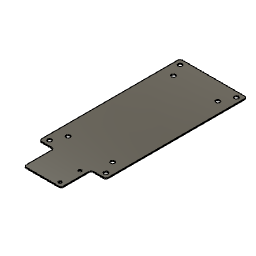
GAD Mount Plane v1 (Autodesk Fusion 360 design; units mm, degrees)
Autodesk Fusion 360 part; units mm, degrees
sketch "Sketch1" plane through (0, 0, 0) normal (0, 0, 1) x (1, 0, 0)
  line L0 (45, 95) -> (-45, 95)
  line L1 (-45, 95) -> (-45, -95)
  line L2 (-45, -95) -> (45, -95)
  line L3 (45, -95) -> (45, 95)
  line L4 (45, 95) -> (-45, -95) construction
  line L5 (-45, 95) -> (45, -95) construction
  line L6 (30, 71) -> (-30, 71) construction
  line L7 (-30, 71) -> (-30, -71) construction
  line L8 (-30, -71) -> (30, -71) construction
  line L9 (30, -71) -> (30, 71) construction
  line L10 (30, 71) -> (-30, -71) construction
  line L11 (-30, 71) -> (30, -71) construction
  circle A0 centre (-30, 71) radius 2.75
  circle A1 centre (30, 71) radius 2.75
  circle A2 centre (-30, -71) radius 2.75
  circle A3 centre (30, -71) radius 2.75
  line L12 (38, 88) -> (-38, 88) construction
  line L13 (-38, 88) -> (-38, -88) construction
  line L14 (-38, -88) -> (38, -88) construction
  line L15 (38, -88) -> (38, 88) construction
  line L16 (38, 88) -> (-38, -88) construction
  line L17 (-38, 88) -> (38, -88) construction
  circle A4 centre (38, 88) radius 2.75
  circle A5 centre (-38, 88) radius 2.75
  circle A6 centre (-38, -88) radius 2.75
  circle A7 centre (38, -88) radius 2.75
  line L18 (-25, -95) -> (25, -95)
  line L19 (25, -95) -> (25, -135.5)
  line L20 (25, -135.5) -> (-25, -135.5)
  line L21 (-25, -135.5) -> (-25, -95)
  line L22 (18, -130) -> (18, -103) construction
  circle A8 centre (18, -130) radius 2
  circle A9 centre (18, -103) radius 2
  line L23 (18, -116.5) -> (2.6311, -116.5) construction
  point P0 (0, -95)
  dimension "d1" = 76
  dimension "d2" = 176
  dimension "d3" = 190
  dimension "d4" = 90
  dimension "d5" = 142
  dimension "d6" = 60
  dimension "d7" = 27
  dimension "d8" = 15
  dimension "d9" = 50
  dimension "d12" = 12
  dimension "d13" = 19
  dimension "d14" = 4
  dimension "d15" = 5.5
  constraint horizontal L0
  constraint perpendicular L0 L1
  constraint parallel L0 L2
  constraint parallel L1 L3
  constraint coincident L4 origin
  constraint coincident L5 origin
  constraint horizontal L6
  constraint perpendicular L6 L7
  constraint parallel L6 L8
  constraint parallel L7 L9
  constraint coincident L10 origin
  constraint coincident L11 origin
  constraint coincident L6.end L7.start
  constraint coincident L6.start L9.end
  constraint coincident L7.end L8.start
  constraint coincident L8.end L9.start
  constraint horizontal L12
  constraint perpendicular L12 L13
  constraint parallel L12 L14
  constraint parallel L13 L15
  constraint coincident L16 origin
  constraint coincident L17 origin
  constraint coincident L12.start L15.end
  constraint coincident L12.end L13.start
  constraint coincident L13.end L14.start
  constraint coincident L14.end L15.start
  constraint horizontal L18
  constraint vertical L19
  constraint horizontal L20
  constraint vertical L21
  constraint coincident L2 L18.start
  constraint perpendicular L18 L22
  constraint coincident L22.start A8.centre
  constraint coincident L22.end A9.centre
  constraint equal A8 A9
  constraint equal A3 A7
  constraint equal A2 A3
  constraint equal A2 A6
  constraint equal A1 A3
  constraint equal A0 A1
  constraint equal A0 A5
  constraint equal A1 A4
  constraint midpoint L18 P0
  constraint midpoint L2 P0
  constraint midpoint L22 L23.start
  constraint perpendicular L22 L23
  measures "d1" distance of L12.start L12.end
  measures "d2" distance of L12.start L14.end
  measures "d3" distance of L0.start L2.end
  measures "d4" distance of L0.start L0.end
  measures "d5" distance of L6.start L8.end
  measures "d6" distance of L6.start L6.end
  measures "d7" distance of L22.start L22.end
  measures "d8" distance of L14 L22.end
  measures "d9" distance of L19.end L20.end
  measures "d12" distance of L9 L22
  measures "d13" distance of L20 L23
  measures "d14" diameter of A8
  measures "d15" diameter of A7
extrude "Extrude1" add sketch "Sketch1" along normal blind 1.27
fillet "Fillet1" radius 3 8 edges at (-25, -135.5, 0.635) (-25, -95, 0.635) (-45, -95, 0.635) (25, -135.5, 0.635) (25, -95, 0.635) (45, -95, 0.635) (45, 95, 0.635) (-45, 95, 0.635)
